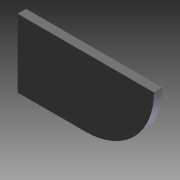
# Autodesk Inventor part: lexan stuff (bottom)
Saved by Autodesk Inventor 2011 (Build 150239000, 239)
## iProperties
Created: 2013-01-27
Part Number: lexan stuff (bottom)
Document SubType Name: Modeling
Designer: Danny
Density: 1 g/cm^3
Author: Danny
Autodesk Inventor part; units mm, degrees
ref_plane "YZ Plane" through (0, 0, 0) normal (1, 0, 0) x (0, 1, 0)
ref_plane "XZ Plane" through (0, 0, 0) normal (0, 1, 0) x (-1, 0, 0)
ref_plane "XY Plane" through (0, 0, 0) normal (0, 0, 1) x (1, 0, 0)
sketch "Sketch1" plane through (0, 0, 0) normal (0, 0, 1) x (1, 0, 0)
  line L0 (-50.8, 0) -> (-101.6, 0)
  line L1 (-101.6, 0) -> (-101.6, 50.8)
  line L2 (-101.6, 50.8) -> (0, 50.8)
  line L3 (0, 50.8) -> (0, 50.8)
  arc A0 (-50.8, 0) -> (0, 50.8) centre (-50.8, 50.8) ccw
  point P0 (0, 0)
  dimension "d0" = 101.6
  dimension "d1" = 50.8
  dimension "d4" = 50.8
  constraints: 8 end point, 2 parallel, 2 point on circle, 2 point on line, 2 tangent, 1 centre point, 1 horizontal, 1 perpendicular
  measures "d0" distance of L1.end L2.end
  measures "d1" distance of L0.end L1.end
  measures "d4" radius of A0
extrude "Extrusion1" add sketch "Sketch1" along normal blind 6.35
body "Solid1"
